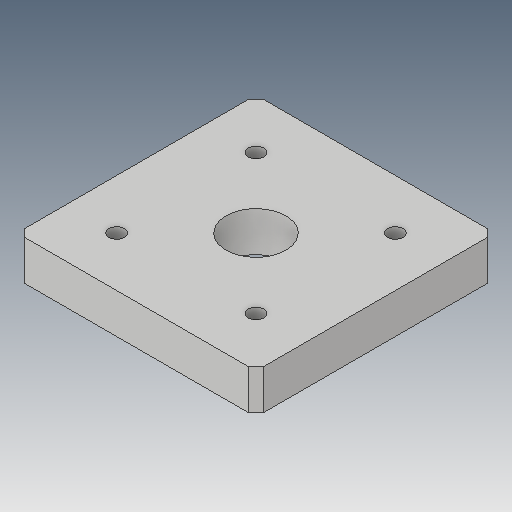
# Autodesk Inventor part: 00_XY_stage-CHUO_SEIKI_LD-647-R1-Top
Saved by Autodesk Inventor 2019 (Build 230136000, 136)
## iProperties
Created: 2019-05-02
Part Number: 00_XY_stage-CHUO_SEIKI_LD-647-R1-Top
Material: Generic
Document SubType Name: Modeling
Designer: diederichbenedict
Density: 1 g/cm^3
Appearance: Default
Author: diederichbenedict
Autodesk Inventor part; units mm, degrees
ref_plane "YZ Plane" through (0, 0, 0) normal (1, 0, 0) x (0, 1, 0)
ref_plane "XZ Plane" through (0, 0, 0) normal (0, 1, 0) x (-1, 0, 0)
ref_plane "XY Plane" through (0, 0, 0) normal (0, 0, 1) x (1, 0, 0)
sketch "Sketch1" plane through (0, 0, 0) normal (0, 1, 0) x (-1, 0, 0)
  line L0 (-30, -30) -> (30, -30)
  line L1 (30, -30) -> (30, 30)
  line L2 (30, 30) -> (-30, 30)
  line L3 (-30, 30) -> (-30, -30)
  line L4 (-30, -30) -> (30, 30) construction
  line L5 (30, -30) -> (-30, 30) construction
  circle A0 centre (0, 0) radius 7.5
  dimension "d0" = 60
  dimension "d1" = 60
  dimension "d13" = 15
  constraints: 12 end point, 2 midpoint, 2 parallel, 1 centre point, 1 coincident, 1 horizontal, 1 perpendicular
  measures "d0" distance of L2.end L1.end
  measures "d1" distance of L1.end L0.end
  measures "d13" diameter of A0
extrude "Extrusion1" add sketch "Sketch1" along normal blind 10
sketch "Sketch2" plane through (0, 10, 0) normal (0, 1, 0) x (1, 0, 0)
  line L0 (30, 30) -> (-30, 30) projected
  line L1 (-30, 30) -> (-30, -30) projected
  line L2 (-30, -30) -> (30, -30) projected
  line L3 (30, -30) -> (30, 30) projected
  line L4 (17.5, -17.5) -> (-17.5, -17.5)
  line L5 (-17.5, -17.5) -> (-17.5, 17.5)
  line L6 (-17.5, 17.5) -> (17.5, 17.5)
  line L7 (17.5, 17.5) -> (17.5, -17.5)
  line L8 (17.5, -17.5) -> (-17.5, 17.5) construction
  line L9 (-17.5, -17.5) -> (17.5, 17.5) construction
  line L10 (0, -17.5) -> (0, 17.5)
  line L11 (-17.5, 0) -> (17.5, 0)
  point P0 (0, 0)
  dimension "d4" = 35
  dimension "d5" = 35
  constraints: 16 end point, 6 midpoint, 2 parallel, 1 horizontal, 1 perpendicular
  measures "d4" distance of L5.end L6.end
  measures "d5" distance of L4.end L5.end
hole "Hole1" at (-17.5, 10, 17.5) at (-17.5, 10, -17.5) at (17.5, 10, -17.5) at (17.5, 10, 17.5) direction (0, -1, 0) diameter 3.9 depth 10 tip angle 118
chamfer "Chamfer1" distance 2 angle 45 4 edges at (30, 5, 30) (30, 5, -30) (-30, 5, -30) (-30, 5, 30)
body "Solid1"
